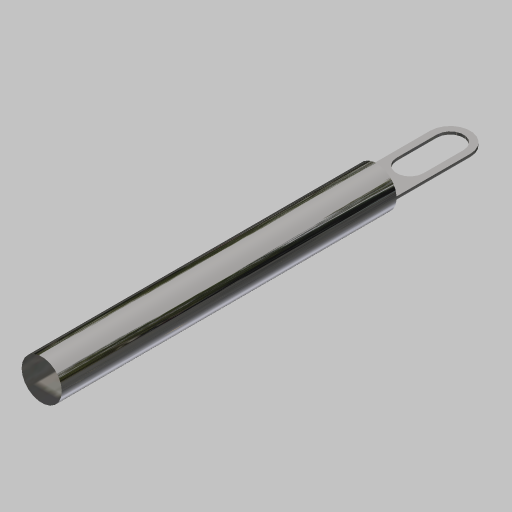
# Autodesk Inventor part: FishHolder
Saved by Autodesk Inventor 2023 (Build 270158000, 158)
## iProperties
Created: 2014-07-16
Part Number: FishHolder
Material: Edelstahl
Document SubType Name: Modeling
Designer: splath
Density: 1 g/cm^3
Appearance: Halbpoliert
Author: splath
Autodesk Inventor part; units mm, degrees
ref_plane "YZ Plane" through (0, 0, 0) normal (1, 0, 0) x (0, 1, 0)
ref_plane "XZ Plane" through (0, 0, 0) normal (0, 1, 0) x (-1, 0, 0)
ref_plane "XY Plane" through (0, 0, 0) normal (0, 0, 1) x (1, 0, 0)
sketch "Skizze1" plane through (0, 0, 0) normal (0, 1, 0) x (-1, 0, 0)
  circle A0 centre (0, 0) radius 1.5
  dimension "d0" = 3
  constraints: 1 centre point, 1 coincident
  measures "d0" diameter of A0
extrude "Extrusion1" add sketch "Skizze1" along normal blind 32
sketch "Skizze2" plane through (0, 0, 0) normal (1, 0, 0) x (0, 1, 0)
  line L0 (32, 1.5) -> (25, 1.5)
  line L1 (25, 1.5) -> (25, 0.1)
  line L2 (25, 0.1) -> (32, 0.1)
  line L3 (32, 0.1) -> (32, -0.1)
  line L4 (32, -0.1) -> (25, -0.1)
  line L5 (25, -0.1) -> (25, -1.5)
  line L6 (25, -1.5) -> (33, -1.5)
  line L7 (33, -1.5) -> (33, 1.5)
  line L8 (33, 1.5) -> (32, 1.5)
  line L9 (32, -1.5) -> (32, 1.5) projected
  line L10 (0, 1.5) -> (0, -1.5) projected
  point P0 (0, 0)
  dimension "d3" = 7
  dimension "d4" = 1.4
  dimension "d5" = 7
  dimension "d6" = 0.2
  dimension "d7" = 7
  dimension "d8" = 1.4
  dimension "d9" = 8
  dimension "d10" = 3
  dimension "d18" = 7
  constraints: 18 end point, 5 perpendicular, 2 parallel, 1 horizontal
  measures "d3" distance of L0.start L0.end
  measures "d4" distance of L0.end L1.end
  measures "d5" distance of L1.end L2.end
  measures "d6" distance of L2.end L3.end
  measures "d7" distance of L3.end L4.end
  measures "d8" distance of L4.end L5.end
  measures "d9" distance of L5.end L6.end
  measures "d10" distance of L6.end L7.end
  measures "d18" distance between parallel lines of L9 L1
extrude "Extrusion2" cut sketch "Skizze2" along normal through all both and the other way through all
fillet "Rundung1" radius 1.5 2 edges at (-1.4992, 32, 0.05) (-1.4992, 32, -0.05)
sketch "Skizze3" plane through (-1.4967, 25, 0.1) normal (0, 0, 1) x (1, 0, 0)
  arc A0 (2.9933, 5.5) -> (0, 5.5) centre (1.4967, 5.5) ccw projected
  line L0 (0, 0) -> (0, 5.5) projected
  line L1 (1.4967, 5.5) -> (1.4967, 2.5) construction
  line L2 (0.4967, 5.5) -> (0.4967, 2.5)
  line L3 (2.4967, 2.5) -> (2.4967, 5.5)
  arc A1 (2.4967, 5.5) -> (0.4967, 5.5) centre (1.4967, 5.5) ccw
  arc A2 (0.4967, 2.5) -> (2.4967, 2.5) centre (1.4967, 2.5) ccw
  point P0 (1.4967, -25)
  point P1 (1.4967, 4)
  dimension "d14" = 3
  dimension "d15" = 2
  constraints: 8 end point, 4 point on circle, 4 tangent, 2 centre point, 2 parallel, 1 midpoint
  measures "d14" distance of L1.start L1.end
  measures "d15" diameter of A2
extrude "Extrusion3" cut sketch "Skizze3" against normal through all
